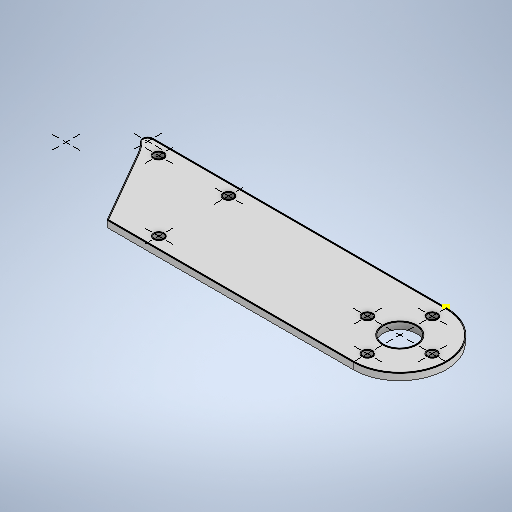
# Autodesk Inventor part: CAM_axis_2_4_connector_frame_non_powered
Saved by Autodesk Inventor 2025.2 (Build 292293000, 293)
## iProperties
Created: 2025-08-09
Part Number: CAM_axis_2_4_connector_frame_non_powered
Material: Generic
Document SubType Name: Modeling
Designer: User
Density: 1 g/cm^3
Appearance: Default
Author: User
Autodesk Inventor part; units mm, degrees
ref_plane "YZ Plane" through (0, 0, 0) normal (1, 0, 0) x (0, 1, 0)
ref_plane "XZ Plane" through (0, 0, 0) normal (0, 1, 0) x (-1, 0, 0)
ref_plane "XY Plane" through (0, 0, 0) normal (0, 0, 1) x (1, 0, 0)
sketch "Sketch1" plane through (0, 0, 0) normal (0, 1, 0) x (-1, 0, 0)
  circle A0 centre (59.6, 2.475) radius 1.05
  circle A1 centre (44.5, 17.525) radius 1.05
  circle A2 centre (44.5, 2.475) radius 1.05
  circle A3 centre (0, 10) radius 3.6
  circle A4 centre (0, 3) radius 1.05
  circle A5 centre (7, 10) radius 1.05
  circle A6 centre (0, 17) radius 1.05
  circle A7 centre (-7, 10) radius 1.05
  line L0 (62.1407, 4.25) -> (53.0474, 20)
  line L1 (0, 20) -> (53.0474, 20)
  arc A8 (62.1407, 4.25) -> (64.1193, 1.72) centre (72.1, 10) ccw
  arc A9 (0, 20) -> (0, 0) centre (0, 10) ccw
  line L2 (63.4253, 0) -> (0, 0)
  arc A10 (63.4253, 0) -> (64.1193, 1.72) centre (63.4253, 1) ccw
  point P0 (0, 0)
  constraints: 11 centre point, 6 end point, 6 equal radius, 6 point on circle, 5 tangent, 2 horizontal, 1 parallel, 28 other
extrude "Extrusion1" add sketch "Sketch1" against normal blind 1.5
body "Solid1"
